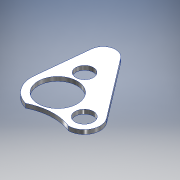
# Autodesk Inventor part: Motor Plate
Saved by Autodesk Inventor 2019.4 (Build 234330000, 330)
## iProperties
Created: 2019-11-30
Part Number: Motor Plate
Material: Aluminum 6061
Document SubType Name: Modeling
Designer: admin
Density: 2.7 g/cm^3
Appearance: Aluminum - Flat
Author: admin
Autodesk Inventor part; units mm, degrees
ref_plane "YZ Plane" through (0, 0, 0) normal (1, 0, 0) x (0, 1, 0)
ref_plane "XZ Plane" through (0, 0, 0) normal (0, 1, 0) x (-1, 0, 0)
ref_plane "XY Plane" through (0, 0, 0) normal (0, 0, 1) x (1, 0, 0)
sketch "Sketch1" plane through (0, 0, 0) normal (0, 1, 0) x (-1, 0, 0)
  circle A0 centre (0, 0) radius 11
  circle A1 centre (-35.6597, 54.0362) radius 11
  line L0 (-35.6597, 54.0362) -> (0, 0) construction
  circle A2 centre (2.7271, 36.9124) radius 23.5
  line L1 (2.7271, 36.9124) -> (0, 0) construction
  line L2 (2.7271, 36.9124) -> (-35.6597, 54.0362) construction
  arc A3 (-53.1131, 46.5277) -> (-22.7141, 67.9434) centre (-35.6597, 54.0362) ccw construction
  arc A4 (16.187, 65.3919) -> (32.9028, 27.8749) centre (2.7271, 36.9124) ccw construction
  arc A5 (14.7055, -32.8848) -> (-18.1343, -34.7797) centre (-2.0588, -27.864) ccw construction
  line L3 (14.7055, -32.8848) -> (32.9028, 27.8749)
  line L4 (-53.1131, 46.5277) -> (-18.1343, -34.7797)
  arc A6 (-22.7141, 67.9434) -> (-53.1131, 46.5277) centre (-35.6597, 54.0362) ccw
  arc A7 (32.9028, 27.8749) -> (16.187, 65.3919) centre (2.7271, 36.9124) ccw
  arc A8 (-18.1343, -34.7797) -> (14.7055, -32.8848) centre (-2.0588, -27.864) ccw
  arc A9 (-22.7141, 67.9434) -> (16.187, 65.3919) centre (0.0245, 116.7976) ccw
  circle A10 centre (-2.0588, -27.864) radius 7.5 construction
  circle A11 centre (-2.0588, -27.864) radius 23.3732 projected
  dimension "d0" = 22
  dimension "d1" = 22
  dimension "d2" = 64.742
  dimension "d3" = 47
  dimension "d4" = 37.013
  dimension "d5" = 42.033
  dimension "d8" = 35
  dimension "d9" = 8
  dimension "d10" = 8
  constraints: 14 point on circle, 10 centre point, 10 end point, 5 coincident, 4 tangent
  measures "d0" diameter of A0
  measures "d1" diameter of A1
  measures "d2" distance of L0.start L0.end
  measures "d3" diameter of A2
  measures "d4" distance of L1.start L0.end
  measures "d5" distance of L1.start L0.start
  measures "d8" diameter of A5
  measures "d9" radial gap between concentric circles of A1 A6
  measures "d10" radial gap between concentric circles of A7 A2
extrude "Extrusion1" add sketch "Sketch1" along normal blind 5 contours A0 A11 L4 A6 A9 A7 L3 | A0 A11 L3 A8 L4
fillet "Fillet1" radius 10 2 edges at (-16.187, 2.5, 65.3919) (22.7141, 2.5, 67.9434)
sketch "Sketch2" plane through (0, 5, 0) normal (0, 1, 0) x (1, 0, 0)
  arc A0 (18.1343, 34.7797) -> (-14.7055, 32.8848) centre (2.0588, 27.864) ccw projected
  point P0 (0, 0)
  constraints: 1 coincident
hole "Hole1" at (2.0588, 5, -27.864) direction (0, -1, 0) diameter 24 end through all
body "Solid1"
